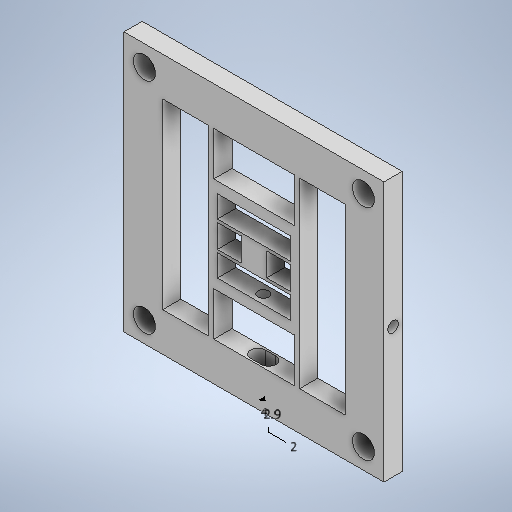
# Autodesk Inventor part: led_holder
Saved by Autodesk Inventor 2025.1 (Build 291241020, 241B)
## iProperties
Created: 2024-10-13
Part Number: led_holder
Material: Ogólny
Document SubType Name: Modeling
Designer: zychlix
Density: 1 g/cm^3
Appearance: Domyślna
Author: zychlix
Autodesk Inventor part; units mm, degrees
ref_plane "YZ Plane" through (0, 0, 0) normal (1, 0, 0) x (0, 1, 0)
ref_plane "XZ Plane" through (0, 0, 0) normal (0, 1, 0) x (-1, 0, 0)
ref_plane "XY Plane" through (0, 0, 0) normal (0, 0, 1) x (1, 0, 0)
sketch "Szkic1" plane through (0, 0, 0) normal (0, 0, 1) x (1, 0, 0)
  line L0 (-35.6, 35.6) -> (35.6, 35.6)
  line L1 (35.6, 35.6) -> (35.6, -35.6)
  line L2 (35.6, -35.6) -> (-35.6, -35.6)
  line L3 (-35.6, -35.6) -> (-35.6, 35.6)
  line L4 (-35.6, -35.6) -> (35.6, 35.6) construction
  line L5 (-35.6, 35.6) -> (35.6, -35.6) construction
  line L6 (-30, 30) -> (30, 30) construction
  line L7 (30, 30) -> (30, -30) construction
  line L8 (30, -30) -> (-30, -30) construction
  line L9 (-30, -30) -> (-30, 30) construction
  circle A0 centre (30, 30) radius 3
  circle A1 centre (30, -30) radius 3
  circle A2 centre (-30, -30) radius 3
  circle A3 centre (-30, 30) radius 3
  circle A4 centre (0, 0) radius 28 construction
  line L10 (-11, 13) -> (11, 13)
  line L11 (-10, 10) -> (10, 10)
  line L12 (10, -10) -> (-10, -10)
  line L13 (-4, 4) -> (4, 4)
  line L14 (3.5, 3.2) -> (3.5, -3.2)
  line L15 (4, -4) -> (-3.8927, -4)
  line L16 (-3.5, -3.2) -> (-3.5, 3.2)
  line L17 (4, 4) -> (10, 4)
  line L18 (-4, 4) -> (-10, 4)
  line L19 (-3.8927, -4) -> (-10, -4)
  line L20 (4, -4) -> (10, -4)
  line L21 (-3.5, 3.2) -> (-10, 3.2)
  line L22 (3.5, 3.2) -> (10, 3.2)
  line L23 (-10, -3.2) -> (-3.5, -3.2)
  line L24 (3.5, -3.2) -> (10, -3.2)
  line L25 (10, 10) -> (10, 4)
  line L26 (-10, 4) -> (-10, 10)
  line L27 (-10, -10) -> (-10, -4)
  line L28 (-10, -3.2) -> (-10, 3.2)
  line L29 (10, 3.2) -> (10, -3.2)
  line L30 (10, -4) -> (10, -10)
  line L31 (-12.5, 12.5) -> (-12.5, 25)
  line L32 (12.5, 12.5) -> (12.5, 25)
  line L33 (11, 13) -> (11, 25)
  line L34 (-11, 13) -> (-11, 25)
  line L35 (-11, 25) -> (11, 25)
  line L36 (-12.5, 25) -> (-25, 25)
  line L37 (-25, 25) -> (-25, 0)
  line L38 (12.5, 25) -> (25, 25)
  line L39 (25, 0) -> (25, 25)
  line L40 (-12.5, 12.5) -> (-12.5, 0)
  line L41 (12.5, 12.5) -> (12.5, 0)
  line L42 (-35.6, 0) -> (35.6, 0) construction
  line L43 (-11, -13) -> (11, -13)
  line L44 (-12.5, -12.5) -> (-12.5, -25)
  line L45 (12.5, -12.5) -> (12.5, -25)
  line L46 (11, -13) -> (11, -25)
  line L47 (-11, -13) -> (-11, -25)
  line L48 (-11, -25) -> (11, -25)
  line L49 (-12.5, -25) -> (-25, -25)
  line L50 (-25, -25) -> (-25, 0)
  line L51 (12.5, -25) -> (25, -25)
  line L52 (25, 0) -> (25, -25)
  line L53 (-12.5, -12.5) -> (-12.5, 0)
  line L54 (12.5, -12.5) -> (12.5, 0)
  point P0 (0, 0)
  point P1 (0, 0)
  dimension "d0" = 60
  dimension "d1" = 35.6
  dimension "d2" = 6
  dimension "d3" = 56
  dimension "d4" = 25
  dimension "d5" = 0.8
  dimension "d6" = 0.8
  dimension "d7" = 20
  dimension "d8" = 7
  dimension "d9" = 6
  dimension "d11" = 1.5
  dimension "d12" = 1.5
  dimension "d13" = 25
  dimension "d14" = 12.5
  dimension "d15" = 12.5
  dimension "d16" = 3
  constraints: 108 end point, 19 point on line, 17 perpendicular, 16 parallel, 10 symmetric about line, 8 horizontal, 6 coincident, 6 vertical, 5 centre point, 4 collinear, 3 equal length, 3 equal radius, 3 midpoint, 12 other
  measures "d0" distance of L6.start L6.end
  measures "d1" distance from line of L3 point (0, 0)
  measures "d2" diameter of A0
  measures "d3" diameter of A4
  measures "d4" distance of L31.start L32.start
  measures "d5" distance between parallel lines of L17 L22
  measures "d6" distance between parallel lines of L20 L24
  measures "d7" distance of L11.start L11.end
  measures "d8" distance between parallel lines of L16 L14
  measures "d9" distance of L11.end L17.end
  measures "d11" distance between parallel lines of L32 L33
  measures "d12" distance between parallel lines of L31 L34
  measures "d13" distance of L36.end L37.end
  measures "d14" distance of L31.end L36.end
  measures "d15" distance of L32.end L38.end
  measures "d16" distance between parallel lines of L11 L10
extrude "Wyciągnięcie proste1" add sketch "Szkic1" along normal blind 5
sketch "Szkic4" plane through (-35.6, -35.6, 0) normal (0, -1, 0) x (1, 0, 0)
  circle A0 centre (35.6506, 2.5) radius 1.45
  circle A1 centre (35.6506, 2.5) radius 2
  line L0 (0, 0) -> (0, 5) construction
  line L1 (0, 2.5) -> (71.3012, 2.5) construction
  line L2 (39.1, 0) -> (39.1, 5) projected
  line L3 (34.2012, 4.5) -> (37.1, 4.5)
  line L4 (39.1, 2.5) -> (39.1, 2.5)
  line L5 (37.1, 0.5) -> (34.2012, 0.5)
  line L6 (32.2012, 2.5) -> (32.2012, 2.5)
  line L7 (32.2012, 4.5) -> (39.1, 0.5) construction
  line L8 (39.1, 4.5) -> (32.2012, 0.5) construction
  arc A2 (39.1, 2.5) -> (37.1, 4.5) centre (37.1, 2.5) ccw
  arc A3 (37.1, 0.5) -> (39.1, 2.5) centre (37.1, 2.5) ccw
  arc A4 (32.2012, 2.5) -> (34.2012, 0.5) centre (34.2012, 2.5) ccw
  arc A5 (34.2012, 4.5) -> (32.2012, 2.5) centre (34.2012, 2.5) ccw
  point P0 (35.6, 0)
  dimension "d19" = 2.9
  dimension "d20" = 4
  dimension "d23" = 2
  constraints: 14 end point, 9 point on line, 8 point on circle, 8 tangent, 6 centre point, 4 midpoint, 3 equal radius, 2 coincident, 2 horizontal, 2 parallel, 1 perpendicular
  measures "d19" diameter of A0
  measures "d20" diameter of A1
  measures "d23" radius of A2
extrude "Wyciągnięcie proste2" cut sketch "Szkic4" against normal blind 26.5 contours A0
extrude "Wyciągnięcie proste3" cut sketch "Szkic4" against normal blind 13 contours A0 | A1 | A1 L3 A2 A3 L5 | A1 L5 A4 A5 L3
sketch "Szkic6" plane through (35.6, -35.6, 0) normal (1, 0, 0) x (0, 0, -1)
  line L0 (0, 71.2) -> (-5, 71.2) construction
  line L1 (-2.5, 71.2) -> (-2.5, 0) construction
  line L2 (0, 0) -> (-5, 0) construction
  circle A0 centre (-2.5, 35.6) radius 1.45
  point P0 (0, 35.6)
  dimension "d26" = 2.9
  constraints: 3 midpoint, 2 end point, 1 centre point
  measures "d26" diameter of A0
extrude "Wyciągnięcie proste4" cut sketch "Szkic6" against normal blind 17
